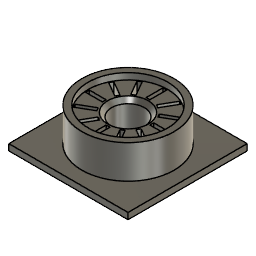
Water Gun Stand - ZURU XSHOT Motor Soaker (Autodesk Fusion 360 archive; units mm, degrees)
design "T-Nut Mounting"
Autodesk Fusion 360 part; units mm, degrees
sketch "Sketch1" plane through (0, 0, 0) normal (0, 0, 1) x (1, 0, 0)
  line L0 (15, 15) -> (-15, 15)
  line L1 (-15, 15) -> (-15, -15)
  line L2 (-15, -15) -> (15, -15)
  line L3 (15, -15) -> (15, 15)
  line L4 (15, 15) -> (-15, -15) construction
  line L5 (-15, 15) -> (15, -15) construction
  dimension "d1" = 30
  dimension "d2" = 30
  constraint horizontal L0
  constraint perpendicular L0 L1
  constraint parallel L0 L2
  constraint parallel L1 L3
  constraint coincident L4 origin
  constraint coincident L5 origin
  measures "d1" distance of L0.start L0.end
  measures "d2" distance of L0.start L2.end
extrude "Extrude1" add sketch "Sketch1" along normal blind 1.6
sketch "Sketch2" plane through (0, 0, 1.6) normal (0, 0, 1) x (-1, 0, 0)
  line L0 (-15, 15) -> (-15, -15)
  line L1 (-15, -15) -> (15, -15)
  line L2 (15, -15) -> (15, 15)
  line L3 (15, 15) -> (-15, 15)
  circle A0 centre (0, 0) radius 11.6
  circle A1 centre (0, 0) radius 10
  circle A2 centre (0, 0) radius 4.1
  dimension "d5" = 20
  dimension "d6" = 1.6
  dimension "d7" = 8.2
  constraint coincident A0.centre A1.centre
  constraint concentric A0 A1
  constraint concentric A1 A2
  measures "d5" diameter of A1
  measures "d6" distance of A0 A1
  measures "d7" diameter of A2
extrude "Extrude2" cut sketch "Sketch2" against normal blind 1.6 contours A2
extrude "Extrude3" add sketch "Sketch2" along normal blind 6.8 contours A1
extrude "Extrude4" add sketch "Sketch2" along normal blind 8.4 contours A0
chamfer "Chamfer1" distance 1 angle 45 1 edges at (3.8225, -1.4826, 8.4)
sketch "Sketch3" plane through (0, 0, 8.4) normal (0, 0, 1) x (-1, 0, 0)
  circle A0 centre (0, 0) radius 10
  circle A1 centre (0, 0) radius 5.1
  line L0 (0, 0) -> (0, 15) construction
  line L1 (0, 5.5) -> (-0.95, 5.5)
  line L2 (-0.95, 5.5) -> (-0.95, 9.75)
  line L3 (-0.95, 9.75) -> (0, 9.75)
  line L4 (0, 9.75) -> (0, 5.5)
  line L5 (15, 15) -> (-15, 15)
  dimension "d15" = 0.95
  dimension "d16" = 4.25
  dimension "d17" = 5.5
  constraint coincident A0.centre A1.centre
  constraint vertical L0
  constraint horizontal L1
  constraint vertical L2
  constraint horizontal L3
  constraint vertical L4
  constraint coincident L0 L1.start
  constraint coincident L0.end L5
  measures "d15" distance of L2.end L3.end
  measures "d16" distance of L1.start L3.end
  measures "d17" distance of A0.centre L1.start
extrude "Extrude5" cut sketch "Sketch3" against normal blind 4.4 contours L1 L2 L3 L4
pattern_circular "C-Pattern1" count 12 over 360 about axis through (0, 0, 8.4) along (0, 0, -1) of "Extrude5"
equation "d2 = d1"
equation "d12 = 6.8 mm + 1.6 mm"
